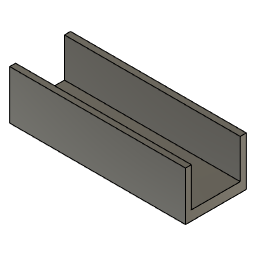
simple_mount_3 v2 (Autodesk Fusion 360 design; units mm, degrees)
Autodesk Fusion 360 part; units mm, degrees
sketch "Sketch1" plane through (0, 0, 0) normal (0, 0, 1) x (1, 0, 0) in component "Mount"
  line L0 (0, 0) -> (89.85, 0)
  line L1 (89.85, 0) -> (89.85, 31.11)
  line L2 (89.85, 31.11) -> (0, 31.11)
  line L3 (0, 31.11) -> (0, 0)
  dimension "d1" = 89.85
  dimension "d2" = 31.11
  constraint horizontal L0
  constraint vertical L1
  constraint horizontal L2
  constraint vertical L3
  constraint coincident L0.start L3.end
  measures "d1" distance of L0.start L0.end
  measures "d2" distance of L0.start L2.end
extrude "Extrude1" add sketch "Sketch1" along normal blind 5 in component "Mount"
sketch "Sketch2" plane through (0, 0, 5) normal (0, 0, 1) x (-1, 0, 0) in component "Mount"
  line L0 (0, -31.11) -> (0, 0)
  line L1 (0, 0) -> (-89.85, 0)
  line L2 (-89.85, 0) -> (-89.85, -31.11)
  line L3 (-89.85, -31.11) -> (0, -31.11)
  line L4 (-44.925, -31.11) -> (-44.925, -28.11) construction
  line L5 (-44.925, 0) -> (-44.925, -3) construction
  line L6 (0, -3) -> (-89.85, -3)
  line L7 (0, -28) -> (-89.85, -28)
  dimension "d5" = 3
  dimension "d6" = 3
  constraint midpoint L3 L4.start
  constraint perpendicular L3 L4
  constraint midpoint L1 L5.start
  constraint perpendicular L1 L5
  constraint coincident L0 L6.start
  constraint coincident L2 L6.end
  constraint perpendicular L2 L6
  constraint coincident L0 L7.start
  constraint coincident L2 L7.end
  constraint perpendicular L2 L7
  measures "d5" distance of L4.start L4.end
  measures "d6" distance of L5.start L5.end
extrude "Extrude2" add sketch "Sketch2" along normal blind 20 contours L0 L2 L3 L7 | L0 L1 L2 L6 in component "Mount"
sketch "Sketch3" plane through (0, 0, 5) normal (0, 0, 1) x (-1, 0, 0) in component "Mount"
  line L0 (0, -3) -> (-89.85, -3)
  line L1 (-89.85, -3) -> (-89.85, -28)
  line L2 (-89.85, -28) -> (0, -28)
  line L3 (0, -28) -> (0, -3)
  line L4 (-44.925, -28) -> (-44.925, -3) construction
  line L5 (-89.85, -15.5) -> (0, -15.5) construction
  line L6 (-44.925, -15.5) -> (-63.425, -15.5) construction
  line L7 (-44.925, -15.5) -> (-26.425, -15.5) construction
  line L8 (-63.425, -15.5) -> (-59.425, -15.5) construction
  line L9 (-26.425, -15.5) -> (-30.425, -15.5) construction
  circle A0 centre (-30.425, -15.5) radius 4 construction
  circle A1 centre (-59.425, -15.5) radius 4 construction
  line L10 (0, -15.5) -> (-21, -15.5) construction
  line L11 (-21, -15.5) -> (-22.25, -15.5) construction
  circle A2 centre (-22.25, -15.5) radius 1.25
  line L12 (-23.5, -15.5) -> (-68.5, -15.5) construction
  line L13 (-68.5, -15.5) -> (-69.75, -15.5) construction
  circle A3 centre (-69.75, -15.5) radius 1.25
  circle A4 centre (-30.425, -15.5) radius 2
  circle A5 centre (-59.425, -15.5) radius 2
  dimension "d9" = 18.5
  dimension "d10" = 18.5
  dimension "d11" = 4
  dimension "d12" = 4
  dimension "d13" = 8
  dimension "d14" = 8
  dimension "d15" = 21
  dimension "d16" = 1.25
  dimension "d17" = 2.5
  dimension "d18" = 45
  dimension "d19" = 1.25
  dimension "d20" = 2.5
  dimension "d21" = 4
  dimension "d22" = 4
  constraint midpoint L2 L4.start
  constraint midpoint L0 L4.end
  constraint midpoint L1 L5.start
  constraint midpoint L3 L5.end
  constraint midpoint L5 L6.start
  constraint perpendicular L4 L6
  constraint perpendicular L4 L7
  constraint parallel L5 L8
  constraint perpendicular L4 L9
  constraint coincident L9.end A0.centre
  constraint coincident L8.end A1.centre
  constraint perpendicular L3 L10
  constraint parallel L5 L11
  constraint coincident L11.end A2.centre
  constraint coincident A2 L12.start
  constraint coincident L5 L12.start
  constraint parallel L7 L12
  constraint parallel L5 L13
  constraint coincident L13.end A3.centre
  measures "d9" distance of L6.start L6.end
  measures "d10" distance of L6.start L7.end
  measures "d11" distance of L6.end L8.end
  measures "d12" distance of L7.end L9.end
  measures "d13" diameter of A0
  measures "d14" diameter of A1
  measures "d15" distance of L5.end L10.end
  measures "d16" distance of L10.end L11.end
  measures "d17" diameter of A2
  measures "d18" distance of L12.start L12.end
  measures "d19" distance of L12.end L13.end
  measures "d20" diameter of A3
  measures "d21" diameter of A4
  measures "d22" diameter of A5
extrude "Extrude3" cut sketch "Sketch3" against normal blind 5 contours A2 | A3 | A4 | A5 in component "Mount"
component "Mount" placed x (1, 0, 0) y (0, 1, 0) z (0, 0, 1) at (0, 0, 0)
